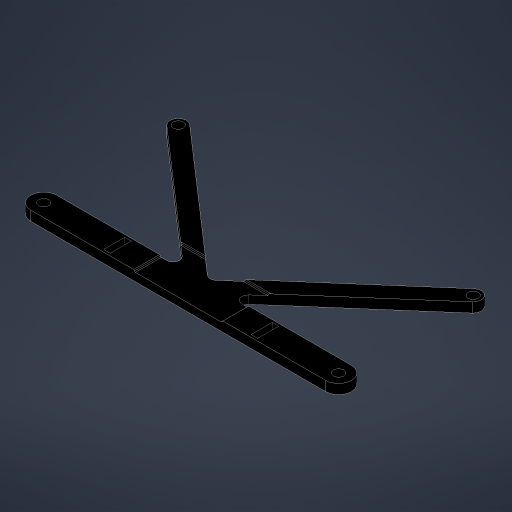
# Autodesk Inventor part: Verstärker
Saved by Autodesk Inventor 2023 (Build 270158000, 158)
## iProperties
Created: 2023-02-27
Part Number: Verstärker
Material: Generic
Document SubType Name: Modeling
Designer: Elias Braun
Density: 1 g/cm^3
Appearance: Default
Author: Elias Braun
Autodesk Inventor part; units mm, degrees
ref_plane "YZ Plane" through (0, 0, 0) normal (1, 0, 0) x (0, 1, 0)
ref_plane "XZ Plane" through (0, 0, 0) normal (0, 1, 0) x (-1, 0, 0)
ref_plane "XY Plane" through (0, 0, 0) normal (0, 0, 1) x (1, 0, 0)
sketch "Sketch2" plane through (0, 0, 0) normal (0, 1, 0) x (-1, 0, 0)
  circle A0 centre (45.4935, -20.7447) radius 1.6
  circle A1 centre (20.7447, -45.4935) radius 1.6
  line L0 (45.4935, -20.7447) -> (20.7447, -45.4935) construction
  line L1 (45.4935, -20.7447) -> (20.7447, -45.4935) construction
  circle A2 centre (20.7447, 45.4935) radius 1.6
  circle A3 centre (45.4935, 20.7447) radius 1.6
  line L2 (20.7447, 45.4935) -> (45.4935, 20.7447) construction
  line L3 (20.7447, 45.4935) -> (45.4935, 20.7447) construction
  circle A4 centre (-45.4935, 20.7447) radius 1.6
  circle A5 centre (-20.7447, 45.4935) radius 1.6
  line L4 (-45.4935, 20.7447) -> (-20.7447, 45.4935) construction
  line L5 (-45.4935, 20.7447) -> (-20.7447, 45.4935) construction
  circle A6 centre (-20.7447, -45.4935) radius 1.6
  circle A7 centre (-45.4935, -20.7447) radius 1.6
  line L6 (-20.7447, -45.4935) -> (-45.4935, -20.7447) construction
  line L7 (-20.7447, -45.4935) -> (-45.4935, -20.7447) construction
  line L8 (45.4935, 24.7447) -> (-45.4935, 24.7447)
  arc A8 (45.4935, 16.7447) -> (45.4935, 24.7447) centre (45.4935, 20.7447) ccw
  arc A9 (-45.4935, 24.7447) -> (-45.4935, 16.7447) centre (-45.4935, 20.7447) ccw
  line L9 (-45.4935, 16.7447) -> (-11.6124, 16.7447)
  line L10 (0, 20.7447) -> (45.4935, 20.7447) construction
  line L11 (0, 20.7447) -> (-45.4935, 20.7447) construction
  line L12 (0, 20.7447) -> (45.4935, -20.7447) construction
  line L13 (1.3139, 14.4336) -> (43.8512, -22.6296)
  arc A10 (43.8512, -22.6296) -> (47.1358, -18.8599) centre (45.4935, -20.7447) ccw
  line L14 (0, 20.7447) -> (-45.4935, -20.7447) construction
  line L15 (-10.2985, 13.2368) -> (-47.1358, -18.8599)
  line L16 (-43.8512, -22.6296) -> (-1.3139, 14.4336)
  arc A11 (-47.1358, -18.8599) -> (-43.8512, -22.6296) centre (-45.4935, -20.7447) ccw
  line L17 (11.6124, 16.7447) -> (45.4935, 16.7447)
  line L18 (47.1358, -18.8599) -> (10.2985, 13.2368)
  arc A12 (11.6124, 16.7447) -> (10.2985, 13.2368) centre (11.6124, 14.7447) ccw
  arc A13 (-10.2985, 13.2368) -> (-11.6124, 16.7447) centre (-11.6124, 14.7447) ccw
  arc A14 (1.3139, 14.4336) -> (-1.3139, 14.4336) centre (0, 12.9257) ccw
  line L19 (23.7467, 23.9947) -> (23.7467, 17.4947)
  line L20 (23.7467, 17.4947) -> (21.7467, 17.4947)
  line L21 (21.7467, 17.4947) -> (21.7467, 23.9947)
  line L22 (21.7467, 23.9947) -> (23.7467, 23.9947)
  line L23 (23.7467, 23.9947) -> (21.7467, 17.4947) construction
  line L24 (23.7467, 17.4947) -> (21.7467, 23.9947) construction
  line L25 (0, 20.7447) -> (0, 17.7311) construction
  line L26 (-23.7467, 23.9947) -> (-23.7467, 17.4947)
  line L27 (-23.7467, 17.4947) -> (-21.7467, 17.4947)
  line L28 (-21.7467, 17.4947) -> (-21.7467, 23.9947)
  line L29 (-21.7467, 23.9947) -> (-23.7467, 23.9947)
  point P0 (26.7551, 33.8262)
  point P1 (-26.7551, 33.8262)
  point P2 (-33.8262, 26.7551)
  point P3 (-33.8262, -26.7551)
  point P4 (-26.7551, -33.8262)
  point P5 (26.7551, -33.8262)
  point P6 (33.8262, -26.7551)
  point P7 (33.8262, 26.7551)
  point P8 (0, 0)
  point P9 (0, 0)
  point P10 (22.7467, 20.7447)
  point P11 (22.7467, 0)
  point P12 (-22.7467, 0)
  dimension "d26" = 360
  dimension "d29" = 8
  dimension "d32" = 5
  dimension "d33" = 5
  dimension "d34" = 2
  dimension "d53" = 6.5
  dimension "d54" = 2
  constraints: 72 end point, 16 tangent, 15 centre point, 14 point on circle, 6 parallel, 5 midpoint, 4 symmetric about line, 2 perpendicular, 1 collinear, 1 equal radius, 1 horizontal, 1 vertical, 26 other
  measures "d29" diameter of A9
  measures "d32" diameter of A10
  measures "d33" diameter of A11
  measures "d34" radius of A12
  measures "d53" distance of L19.start L19.end
  measures "d54" distance of L19.end L20.end
extrude "Extrusion1" add sketch "Sketch2" along normal blind 3 contours A8 L17 A12 L18 A10 L13 A14 L16 A11 L15 A13 L9 A9 L8
sketch "Sketch3" plane through (0, 3, 0) normal (0, 1, 0) x (1, 0, 0)
  circle A0 centre (-45.4935, 20.7447) radius 1.6
  circle A1 centre (-20.7447, 45.4935) radius 1.6
  line L0 (-45.4935, 20.7447) -> (-20.7447, 45.4935) construction
  line L1 (-45.4935, 20.7447) -> (-20.7447, 45.4935) construction
  circle A2 centre (-20.7447, -45.4935) radius 1.6
  circle A3 centre (-45.4935, -20.7447) radius 1.6
  line L2 (-20.7447, -45.4935) -> (-45.4935, -20.7447) construction
  line L3 (-20.7447, -45.4935) -> (-45.4935, -20.7447) construction
  circle A4 centre (45.4935, -20.7447) radius 1.6
  circle A5 centre (20.7447, -45.4935) radius 1.6
  line L4 (45.4935, -20.7447) -> (20.7447, -45.4935) construction
  line L5 (45.4935, -20.7447) -> (20.7447, -45.4935) construction
  circle A6 centre (20.7447, 45.4935) radius 1.6
  circle A7 centre (45.4935, 20.7447) radius 1.6
  line L6 (20.7447, 45.4935) -> (45.4935, 20.7447) construction
  line L7 (20.7447, 45.4935) -> (45.4935, 20.7447) construction
  line L8 (-45.4935, -23.2447) -> (45.4935, -23.2447)
  arc A8 (-45.4935, -18.2447) -> (-45.4935, -23.2447) centre (-45.4935, -20.7447) ccw
  arc A9 (45.4935, -23.2447) -> (45.4935, -18.2447) centre (45.4935, -20.7447) ccw
  line L9 (45.4935, -18.2447) -> (11.6124, -18.2447)
  line L10 (0, -20.7447) -> (-45.4935, -20.7447) construction
  line L11 (0, -20.7447) -> (45.4935, -20.7447) construction
  line L12 (-25.9967, -21.7447) -> (-19.4967, -21.7447)
  line L13 (-19.4967, -21.7447) -> (-19.4967, -19.7447)
  line L14 (-19.4967, -19.7447) -> (-25.9967, -19.7447)
  line L15 (-25.9967, -19.7447) -> (-25.9967, -21.7447)
  line L16 (-25.9967, -21.7447) -> (-19.4967, -19.7447) construction
  line L17 (-19.4967, -21.7447) -> (-25.9967, -19.7447) construction
  line L18 (19.4967, -19.7447) -> (25.9967, -19.7447)
  line L19 (19.4967, -21.7447) -> (19.4967, -19.7447)
  line L20 (25.9967, -21.7447) -> (19.4967, -21.7447)
  line L21 (25.9967, -19.7447) -> (25.9967, -21.7447)
  line L22 (0, -20.7447) -> (-45.4935, 20.7447) construction
  line L23 (-1.3477, -16.1321) -> (-43.8089, 22.5919)
  arc A10 (-43.8089, 22.5919) -> (-47.1781, 18.8975) centre (-45.4935, 20.7447) ccw
  line L24 (0, -20.7447) -> (45.4935, 20.7447) construction
  line L25 (10.2647, -14.767) -> (47.1781, 18.8975)
  line L26 (43.8089, 22.5919) -> (1.3477, -16.1321)
  arc A11 (47.1781, 18.8975) -> (43.8089, 22.5919) centre (45.4935, 20.7447) ccw
  line L27 (-2.5, -18.2447) -> (-2.7413, -18.2447)
  line L28 (-11.6124, -18.2447) -> (-45.4935, -18.2447)
  line L29 (-47.1781, 18.8975) -> (-10.2647, -14.767)
  arc A12 (-1.6846, -18.8975) -> (-1.8472, -19.0601) centre (0, -20.7447) ccw
  arc A13 (1.8472, -19.0601) -> (1.6846, -18.8975) centre (0, -20.7447) ccw
  arc A14 (-11.6124, -18.2447) -> (-10.2647, -14.767) centre (-11.6124, -16.2447) ccw
  arc A15 (10.2647, -14.767) -> (11.6124, -18.2447) centre (11.6124, -16.2447) ccw
  arc A16 (-1.3477, -16.1321) -> (1.3477, -16.1321) centre (0, -14.6544) ccw
  line L30 (-13.5, -31.2447) -> (13.5, -31.2447)
  line L31 (13.5, -31.2447) -> (13.5, -10.2447)
  line L32 (13.5, -10.2447) -> (-13.5, -10.2447)
  line L33 (-13.5, -10.2447) -> (-13.5, -31.2447)
  line L34 (-13.5, -31.2447) -> (13.5, -10.2447) construction
  line L35 (13.5, -31.2447) -> (-13.5, -10.2447) construction
  point P0 (26.7551, 33.8262)
  point P1 (-26.7551, 33.8262)
  point P2 (-33.8262, 26.7551)
  point P3 (-33.8262, -26.7551)
  point P4 (-26.7551, -33.8262)
  point P5 (26.7551, -33.8262)
  point P6 (33.8262, -26.7551)
  point P7 (33.8262, 26.7551)
  point P8 (0, 0)
  point P9 (0, 0)
  point P10 (-22.7467, -20.7447)
  point P11 (-22.7467, 0)
  point P12 (22.7467, 0)
  dimension "d40" = 360
  dimension "d41" = 5
  dimension "d42" = 6.5
  dimension "d43" = 2
  dimension "d44" = 5
  dimension "d45" = 5
  dimension "d46" = 2
  dimension "d47" = 2
  dimension "d48" = 27
  dimension "d49" = 21
  constraints: 84 end point, 20 tangent, 18 point on circle, 17 centre point, 9 parallel, 7 midpoint, 3 point on line, 2 perpendicular, 1 collinear, 1 equal radius, 25 other
  measures "d41" diameter of A9
  measures "d42" distance of L12.start L12.end
  measures "d43" distance of L13.end L12.end
  measures "d44" diameter of A10
  measures "d45" diameter of A11
  measures "d46" radius of A14
  measures "d47" radius of A16
  measures "d48" distance of L30.start L30.end
  measures "d49" distance of L31.end L30.end
extrude "Extrusion2" cut sketch "Sketch3" against normal blind 0.5 contours L33 L28 A14 L29 L32 L23 A16 L26 L31 L25 A15 L9 L8 | L8 L31 L30 L33 | L33 L29 A14 L28 | L9 A15 L25 L31 | L32 L26 A16 L23
fillet "Fillet1" radius 0.25 12 edges at (-13.5, 2.5, 20.7447) (-13.5, 3, 20.7447) (-13.5, 2.5, 10.346) (-9.8107, 2.5, 10.2447) (-9.8107, 3, 10.2447) (-13.5, 3, 10.346) (9.8107, 2.5, 10.2447) (9.8107, 3, 10.2447) (13.5, 3, 10.346) (13.5, 2.5, 10.346) (13.5, 2.5, 20.7447) (13.5, 3, 20.7447)
body "Solid1"
